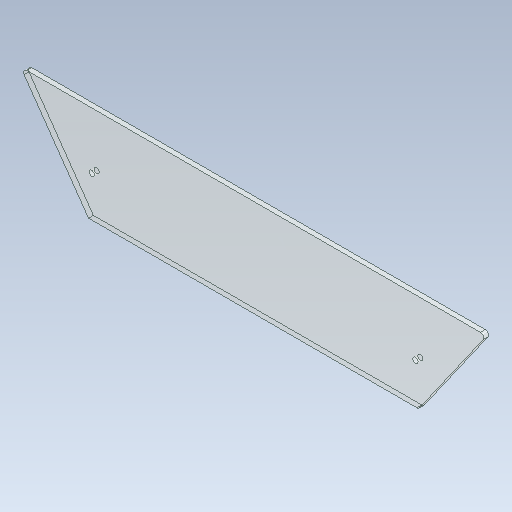
# Autodesk Inventor part: UpperAcrylicSheetBack
Saved by Autodesk Inventor 2021 (Build 250183000, 183)
## iProperties
Created: 2020-07-17
Part Number: UpperAcrylicSheetBack
Material: Generic
Document SubType Name: Modeling
Designer: CASE-SMALL2
Density: 1 g/cm^3
Appearance: Default
Author: CASE-SMALL2
Autodesk Inventor part; units mm, degrees
ref_plane "YZ Plane" through (0, 0, 0) normal (1, 0, 0) x (0, 1, 0)
ref_plane "XZ Plane" through (0, 0, 0) normal (0, 1, 0) x (-1, 0, 0)
ref_plane "XY Plane" through (0, 0, 0) normal (0, 0, 1) x (1, 0, 0)
sketch "Sketch1" plane through (0, 0, 0) normal (0, 0, 1) x (1, 0, 0)
  line L0 (-144, -30) -> (144, -30)
  line L1 (144, -30) -> (144, 30)
  line L2 (144, 30) -> (-144, 30)
  line L3 (-144, 30) -> (-144, -30)
  line L4 (-144, -30) -> (144, 30) construction
  line L5 (144, -30) -> (-144, 30) construction
  line L6 (144, 30) -> (101.9875, -30)
  line L7 (-144, 30) -> (-101.9875, -30)
  point P0 (0, 0)
  dimension "d0" = 288
  dimension "d1" = 60
  dimension "d2" = 55
  dimension "d13" = 55
  constraints: 16 end point, 2 midpoint, 2 parallel, 2 point on line, 1 horizontal, 1 perpendicular
  measures "d0" distance of L1.end L2.end
  measures "d1" distance of L0.end L1.end
  measures "d2" angle of L0 L6
  measures "d13" angle of L0 L7
extrude "Extrusion1" add sketch "Sketch1" along normal blind 3 contours L7 L2 L6 L0
sketch "Sketch2" plane through (0, 0, 3) normal (0, 0, 1) x (1, 0, 0)
  circle A0 centre (-100, -5) radius 1.65
  line L0 (-101.9875, -30) -> (101.9875, -30) projected
  line L1 (-100, -5) -> (155.6099, -5) construction
  circle A1 centre (100, -5) radius 1.65
  point P0 (0, 0)
  dimension "d5" = 25
  dimension "d6" = 3.3
  dimension "d9" = 3.3
  dimension "d14" = 100
  dimension "d15" = 100
  constraints: 2 centre point, 2 end point, 1 horizontal, 1 point on line
  measures "d5" distance from line of L0 L1.start
  measures "d6" diameter of A0
  measures "d9" diameter of A1
  measures "d14" horizontal distance of point (0, 0) L1.start
  measures "d15" horizontal distance of A1.centre point (0, 0)
extrude "Extrusion2" cut sketch "Sketch2" against normal through all
fillet "Fillet1" radius 2 3 edges at (-144, 30, 1.5) (101.9875, -30, 1.5) (144, 30, 1.5)
sketch "Sketch3" plane through (0, 0, 3) normal (0, 0, 1) x (1, 0, 0)
  arc A0 (141.7963, 26.8528) -> (140.158, 30) centre (140.158, 28) ccw projected
  line L0 (140.158, 30) -> (-140.158, 30) projected
  arc A1 (-140.158, 30) -> (-141.7963, 26.8528) centre (-140.158, 28) ccw projected
  line L1 (-141.7963, 26.8528) -> (-101.9875, -30) projected
  line L2 (-101.9875, -30) -> (100.9464, -30) projected
  arc A2 (100.9464, -30) -> (102.5847, -29.1472) centre (100.9464, -28) ccw projected
  line L3 (102.5847, -29.1472) -> (141.7963, 26.8528) projected
  circle A3 centre (-100, -5) radius 1.65 projected
  circle A4 centre (100, -5) radius 1.65 projected
  point P0 (0, 0)
equation "\"d13\" = d2"
equation "\"d9\" = d6"
equation "\"d15\" = d14"
body "Solid1"
